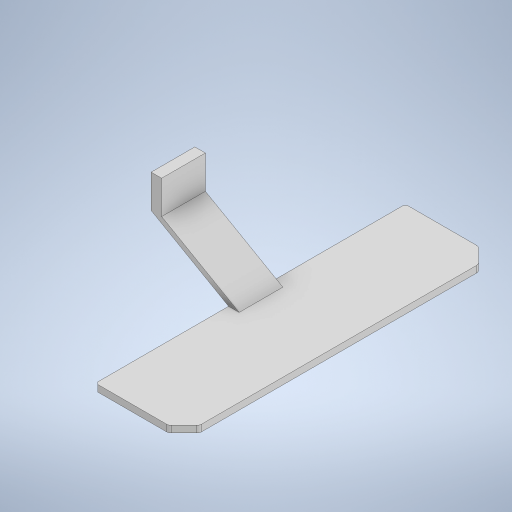
# Autodesk Inventor part: DudukanLineSensor
Saved by Autodesk Inventor 2024 (Build 280153000, 153)
## iProperties
Created: 2025-12-15
Part Number: DudukanLineSensor
Material: Generic
Document SubType Name: Modeling
Designer: risda
Density: 1 g/cm^3
Appearance: Default
Author: risda
Autodesk Inventor part; units mm, degrees
ref_plane "YZ Plane" through (0, 0, 0) normal (1, 0, 0) x (0, 1, 0)
ref_plane "XZ Plane" through (0, 0, 0) normal (0, 1, 0) x (-1, 0, 0)
ref_plane "XY Plane" through (0, 0, 0) normal (0, 0, 1) x (1, 0, 0)
sketch "Sketch1" plane through (0, 0, 0) normal (0, 1, 0) x (-1, 0, 0)
  line L0 (0, 0) -> (0, -19.75)
  line L1 (0, -19.75) -> (-4.75, -19.75)
  line L2 (-4.75, -19.75) -> (-4.75, 0)
  line L3 (-4.75, 0) -> (0, 0)
  dimension "d0" = 19.75
  dimension "d1" = 4.75
  constraints: 8 end point, 3 perpendicular, 1 vertical
  measures "d0" distance of L0.start L0.end
  measures "d1" distance of L0.end L1.end
extrude "Extrusion1" add sketch "Sketch1" along normal blind 15
sketch "Sketch3" plane through (0, 0, 0) normal (0, 0, 1) x (1, 0, 0)
  line L0 (0, 0) -> (0, -60)
  line L1 (4.75, 0) -> (0, 0) projected
  line L2 (0, 0) -> (0, -55)
  line L3 (0, 0) -> (0, -50)
  line L4 (0, 0) -> (35, 0)
  line L5 (4.75, 0) -> (39.75, 0)
  line L6 (0, 0) -> (35, -20)
  line L7 (4.75, 0) -> (39.75, -20)
  line L8 (35, -20) -> (39.75, -20)
  dimension "d4" = 60
  dimension "d5" = 55
  dimension "d6" = 50
  dimension "d7" = 35
  dimension "d8" = 35
  dimension "d23" = 20
  dimension "d24" = 20
  constraints: 16 end point, 3 horizontal, 2 point on line, 1 vertical
  measures "d4" distance of L0.start L0.end
  measures "d5" distance of L0.start L2.end
  measures "d6" distance of L0.start L3.end
  measures "d7" distance of L0.start L4.end
  measures "d8" distance of L1.start L5.end
  measures "d23" vertical distance of L0.start L6.end
  measures "d24" vertical distance of L1.start L7.end
extrude "Extrusion2" add sketch "Sketch3" against normal blind 19.75
sketch "Sketch4" plane through (35, -20, 0) normal (0, -1, 0) x (1, 0, 0)
  line L0 (0, 0) -> (0, -19.75) projected
  line L1 (0, -9.875) -> (0, 60.125)
  line L2 (0, -9.875) -> (0, -79.875)
  line L3 (0, -79.875) -> (40, -79.875)
  line L4 (40, -79.875) -> (40, 60.125)
  line L5 (40, 60.125) -> (0, 60.125)
  point P0 (-35, 0)
  dimension "d11" = 70
  dimension "d12" = 70
  dimension "d13" = 40
  constraints: 10 end point, 2 perpendicular, 2 vertical, 1 horizontal, 1 midpoint
  measures "d11" distance of L1.start L1.end
  measures "d12" distance of L1.start L2.end
  measures "d13" distance of L2.end L3.end
extrude "Extrusion3" add sketch "Sketch4" along normal blind 3
chamfer "Chamfer1" distance 1 angle 45 2 edges at (35, -21.5, 60.125) (35, -21.5, -79.875)
chamfer "Chamfer2" distance 7 angle 45 2 edges at (75, -21.5, 60.125) (75, -21.5, -79.875)
fillet "Fillet1" radius 2 4 edges at (75, -21.5, 53.125) (68, -21.5, 60.125) (75, -21.5, -72.875) (68, -21.5, -79.875)
body "Solid1"
